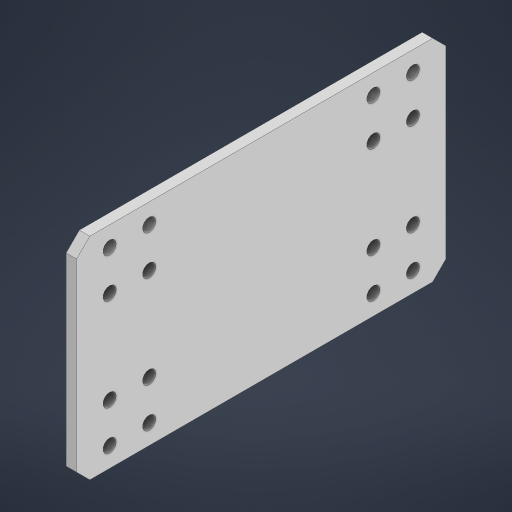
# Autodesk Inventor part: ArmSidePlate
Saved by Autodesk Inventor 2024 (Build 280153000, 153)
## iProperties
Created: 2023-10-25
Part Number: ArmSidePlate
Material: Generic
Document SubType Name: Modeling
Designer: avsar
Density: 1 g/cm^3
Appearance: Default
Author: avsar
Autodesk Inventor part; units mm, degrees
ref_plane "YZ Plane" through (0, 0, 0) normal (1, 0, 0) x (0, 1, 0)
ref_plane "XZ Plane" through (0, 0, 0) normal (0, 1, 0) x (-1, 0, 0)
ref_plane "XY Plane" through (0, 0, 0) normal (0, 0, 1) x (1, 0, 0)
sketch "Sketch1" plane through (0, 0, 0) normal (1, 0, 0) x (0, 1, 0)
  line L0 (-32, 56) -> (32, 56)
  line L1 (32, 56) -> (32, -56)
  line L2 (32, -56) -> (-32, -56)
  line L3 (-32, -56) -> (-32, 56)
  line L4 (-32, 56) -> (32, -56) construction
  line L5 (32, 56) -> (-32, -56) construction
  point P0 (0, 0)
  dimension "d0" = 64
  dimension "d1" = 112
  constraints: 12 end point, 2 midpoint, 2 parallel, 1 horizontal, 1 perpendicular
  measures "d0" distance of L1.end L2.end
  measures "d1" distance of L0.end L1.end
extrude "Extrusion1" add sketch "Sketch1" along normal blind 3.175
sketch "Sketch2" plane through (3.175, 0, 0) normal (1, 0, 0) x (0, 0, -1)
  circle A0 centre (-40, -20) radius 2.5 construction
  line L0 (-56, -32) -> (56, -32) construction
  line L1 (0, -32) -> (0, 32) construction
  line L2 (56, 32) -> (-56, 32) construction
  line L3 (-56, 32) -> (-56, -32) construction
  line L4 (-56, 0) -> (56, 0) construction
  line L5 (56, -32) -> (56, 32) construction
  circle A1 centre (-46, -14) radius 2
  circle A2 centre (-46, -26) radius 2
  circle A3 centre (-34, -26) radius 2
  circle A4 centre (-34, -14) radius 2
  circle A5 centre (-46, 14) radius 2
  circle A6 centre (-46, 26) radius 2
  circle A7 centre (-34, 26) radius 2
  circle A8 centre (-34, 14) radius 2
  circle A9 centre (46, -14) radius 2
  circle A10 centre (46, -26) radius 2
  circle A11 centre (34, -26) radius 2
  circle A12 centre (34, -14) radius 2
  circle A13 centre (46, 14) radius 2
  circle A14 centre (46, 26) radius 2
  circle A15 centre (34, 26) radius 2
  circle A16 centre (34, 14) radius 2
  point P0 (0, 0)
  dimension "d4" = 5
  dimension "d5" = 40
  dimension "d6" = 12
  dimension "d7" = 4
  dimension "d8" = 6
  dimension "d9" = 6
  dimension "d12" = 360
  constraints: 17 centre point, 12 symmetric about line, 4 end point, 4 midpoint, 21 other
  measures "d4" diameter of A0
  measures "d5" horizontal distance of point (0, 0) A0.centre
  measures "d6" distance from line of L0 A0.centre
  measures "d7" diameter of A1
  measures "d8" horizontal distance of A1.centre A0.centre
  measures "d9" horizontal distance of A0.centre A1.centre
extrude "Extrusion2" cut sketch "Sketch2" against normal through all
chamfer "Chamfer1" distance 4 angle 45 2 edges at (1.5875, 32, 56) (1.5875, 32, -56)
chamfer "Chamfer2" distance 4 angle 45 2 edges at (1.5875, -32, 56) (1.5875, -32, -56)
body "Solid1"
